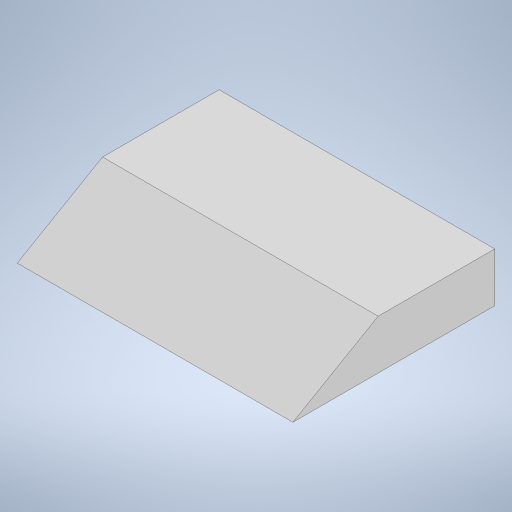
# Autodesk Inventor part: Base
Saved by Autodesk Inventor 2023 (Build 270158000, 158)
## iProperties
Created: 2024-03-02
Part Number: Base
Material: Generic
Document SubType Name: Modeling
Designer: LENOVO
Density: 1 g/cm^3
Appearance: Default
Author: LENOVO
Autodesk Inventor part; units mm, degrees
ref_plane "YZ Plane" through (0, 0, 0) normal (1, 0, 0) x (0, 1, 0)
ref_plane "XZ Plane" through (0, 0, 0) normal (0, 1, 0) x (-1, 0, 0)
ref_plane "XY Plane" through (0, 0, 0) normal (0, 0, 1) x (1, 0, 0)
sketch "Sketch1" plane through (0, 0, 0) normal (0, 1, 0) x (-1, 0, 0)
  line L0 (0, 0) -> (-280, 0)
  line L1 (-280, 0) -> (-280, -205)
  line L2 (-280, -205) -> (0, -205)
  line L3 (0, -205) -> (0, 0)
  dimension "d0" = 280
  dimension "d1" = 205
  constraints: 8 end point, 2 parallel, 1 horizontal, 1 perpendicular
  measures "d0" distance of L2.end L1.end
  measures "d1" distance of L1.end L0.end
extrude "Extrusion1" add sketch "Sketch1" along normal blind 50
sketch "Sketch2" plane through (280, 0, 0) normal (1, 0, 0) x (0, 0, -1)
  line L0 (0, 0) -> (205, 0) projected
  line L1 (0, 0) -> (86.6025, 50)
  line L2 (0, 50) -> (205, 50) projected
  line L3 (0, 0) -> (0, 50) projected
  line L4 (86.6025, 50) -> (0, 50)
  line L5 (0, 50) -> (0, 0)
  dimension "d4" = 100
  constraints: 6 end point, 2 perpendicular, 1 point on line
  measures "d4" distance of L0.start L1.end
extrude "Extrusion2" cut sketch "Sketch2" against normal blind 280
body "Solid1"
